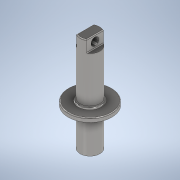
# Autodesk Inventor part: Hydraulic fluid shield
Saved by Autodesk Inventor 2022 (Build 260153000, 153)
## iProperties
Created: 2021-07-24
Part Number: Hydraulic fluid shield
Material: Steel, High Strength, Low Alloy
Document SubType Name: Modeling
Designer: Ian Kibandi
Density: 7.85 g/cm^3
Appearance: Steel - Polished
Author: Ian Kibandi
Autodesk Inventor part; units mm, degrees
ref_plane "YZ Plane" through (0, 0, 0) normal (1, 0, 0) x (0, 1, 0)
ref_plane "XZ Plane" through (0, 0, 0) normal (0, 1, 0) x (-1, 0, 0)
ref_plane "XY Plane" through (0, 0, 0) normal (0, 0, 1) x (1, 0, 0)
sketch "Sketch1" plane through (0, 0, 0) normal (0, 0, 1) x (1, 0, 0)
  line L0 (15, 0) -> (25, 0)
  line L1 (25, 225) -> (0, 225)
  line L2 (0, 225) -> (0, 205)
  line L3 (25, 0) -> (25, 100)
  line L4 (25, 100) -> (50, 100)
  line L5 (50, 100) -> (50, 95)
  line L6 (50, 95) -> (55, 95)
  line L7 (55, 95) -> (55, 103)
  line L8 (53, 105) -> (30, 105)
  line L9 (25, 110) -> (25, 225)
  arc A0 (55, 103) -> (53, 105) centre (53, 103) ccw
  arc A1 (25, 110) -> (30, 105) centre (30, 110) ccw
  line L10 (0, 0) -> (0, 225)
  line L11 (15, 0) -> (15, 200)
  line L12 (10, 205) -> (0, 205)
  arc A2 (15, 200) -> (10, 205) centre (10, 200) ccw
  point P0 (20, 205)
  point P1 (55, 105)
  point P2 (25, 105)
  point P3 (15, 205)
  dimension "d1" = 10
  dimension "d2" = 225
  dimension "d3" = 20
  dimension "d4" = 20
  dimension "d6" = 100
  dimension "d7" = 25
  dimension "d8" = 5
  dimension "d9" = 5
  dimension "d10" = 10
  dimension "d11" = 2
  dimension "d12" = 5
  dimension "d28" = 205
  dimension "d29" = 5
  constraints: 26 end point, 8 perpendicular, 7 point on line, 6 point on circle, 6 tangent, 3 centre point, 2 vertical, 1 collinear
  measures "d1" distance of L0.start L0.end
  measures "d2" distance of L0.end L1.start
  measures "d3" distance of L1.end L2.end
  measures "d4" distance of L2.end point (20, 205)
  measures "d6" distance of L0.end L3.end
  measures "d7" distance of L3.end L4.end
  measures "d8" distance of L4.end L5.end
  measures "d9" distance of L5.end L6.end
  measures "d10" distance of L6.end point (55, 105)
  measures "d11" radius of A0
  measures "d12" radius of A1
  measures "d28" distance of L0.start point (15, 205)
  measures "d29" radius of A2
revolve "Revolution1" add sketch "Sketch1" angle 360 about axis through (0, 0, 0) along (0, 1, 0)
sketch "Sketch2" plane through (0, 225, 0) normal (0, 1, 0) x (1, 0, 0)
  circle A0 centre (0, 0) radius 25 projected
  line L0 (-12.5, 21.6506) -> (-12.5, -21.6506)
  line L1 (12.5, 0) -> (12.5, 21.6506)
  line L2 (12.5, 21.6506) -> (12.5, -21.6506)
  arc A1 (12.5, 21.6506) -> (-12.5, 21.6506) centre (0, 0) ccw
  arc A2 (-12.5, -21.6506) -> (12.5, -21.6506) centre (0, 0) ccw
  dimension "d14" = 12.5
  constraints: 8 point on circle, 6 end point, 2 centre point, 2 coincident, 1 point on line, 1 vertical
  measures "d14" distance of point (0, 0) L1.start
extrude "Extrusion1" add sketch "Sketch2" along normal blind 30 contours L1 L2 A0 L0
sketch "Sketch3" plane through (12.5, 225, 21.6506) normal (1, 0, 0) x (0, 0, -1)
  line L0 (0, 0) -> (43.3013, 0) projected
  line L1 (43.3013, 0) -> (43.3013, 30) projected
  line L2 (0, 30) -> (-3.3494, 30) projected
  circle A0 centre (21.6506, 15) radius 5
  point P0 (21.6506, -225)
  dimension "d18" = 10
  constraints: 1 centre point
  measures "d18" diameter of A0
hole "Hole1" at (12.5, 240, 0) direction (-1, 0, 0) diameter 20 end through all
fillet "Fillet1" radius 2 2 edges at (-12.5, 225, 0) (12.5, 225, -10.8253)
fillet "Fillet2" radius 2 4 edges at (12.5, 255, -10.8253) (-12.5, 255, 0) (0, 255, 25) (0, 255, -25)
body "Solid1"
